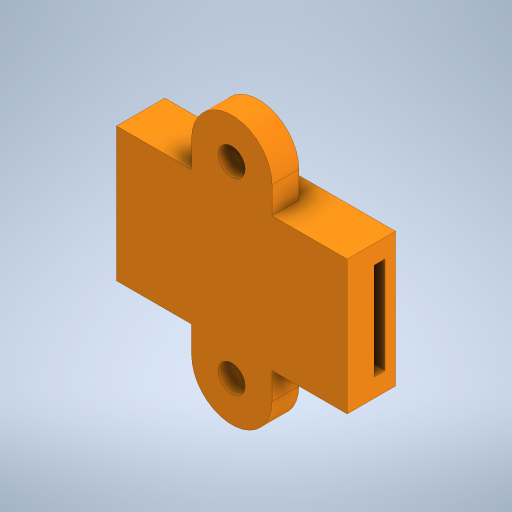
# Autodesk Inventor part: RelayBracket
Saved by Autodesk Inventor 2023 (Build 270158000, 158)
## iProperties
Created: 2022-09-10
Part Number: RelayBracket
Material: Generic
Document SubType Name: Modeling
Designer: Nathann
Density: 1 g/cm^3
Appearance: Orange
Author: Nathann
Autodesk Inventor part; units mm, degrees
ref_plane "YZ Plane" through (0, 0, 0) normal (1, 0, 0) x (0, 1, 0)
ref_plane "XZ Plane" through (0, 0, 0) normal (0, 1, 0) x (-1, 0, 0)
ref_plane "XY Plane" through (0, 0, 0) normal (0, 0, 1) x (1, 0, 0)
sketch "Sketch1" plane through (0, 0, 0) normal (0, 0, 1) x (1, 0, 0)
  line L0 (24.4382, -12.9356) -> (-18.5618, -12.9356)
  line L1 (-18.5618, -12.9356) -> (-18.5618, 12.0644)
  line L2 (-18.5618, 12.0644) -> (24.4382, 12.0644)
  line L3 (24.4382, 12.0644) -> (24.4382, -12.9356)
  line L4 (-4.5618, -12.9356) -> (10.4382, -12.9356)
  line L5 (10.4382, -12.9356) -> (10.4382, -17.9356)
  line L6 (10.4382, -17.9356) -> (-4.5618, -17.9356)
  line L7 (-4.5618, -17.9356) -> (-4.5618, -12.9356)
  line L8 (-4.5618, 12.0644) -> (10.4382, 12.0644)
  line L9 (10.4382, 12.0644) -> (10.4382, 17.0644)
  line L10 (10.4382, 17.0644) -> (-4.5618, 17.0644)
  line L11 (-4.5618, 17.0644) -> (-4.5618, 12.0644)
  circle A0 centre (2.9382, -17.9356) radius 7.5
  circle A1 centre (2.9382, 17.0644) radius 7.5
  circle A2 centre (2.9382, -17.9356) radius 2.5
  circle A3 centre (2.9382, 17.0644) radius 2.5
  point P0 (0, 0)
  point P1 (-4.5618, -17.9356)
  dimension "d0" = 43
  dimension "d1" = 25
  dimension "d2" = 15
  dimension "d3" = 15
  dimension "d4" = 21.5
  dimension "d5" = 21.5
  dimension "d6" = 5
  dimension "d7" = 5
  dimension "d8" = 5
  dimension "d9" = 5
  constraints: 24 end point, 6 parallel, 3 horizontal, 3 perpendicular, 2 centre point, 2 coincident, 2 midpoint, 2 point on line, 6 other
  measures "d0" distance of L0.start L0.end
  measures "d1" distance of L2.end L0.start
  measures "d2" distance between parallel lines of L7 L5
  measures "d3" distance between parallel lines of L11 L9
  measures "d4" distance from line of L1 point (2.938, 17.064)
  measures "d5" distance from line of L1 point (2.938, -17.936)
  measures "d6" distance of L8.end L9.end
  measures "d7" distance of L4.end L5.end
  measures "d8" diameter of A2
  measures "d9" diameter of A3
extrude "Extrusion1" add sketch "Sketch1" along normal blind 5 contours L0 A0 L1 L2 A1 L3 | L5 A0 L0 | A0 L6 A2 L0 | L0 A0 | A0 L6 A2 | L2 A1 L9 | A0 L7 L0 | A1 L2 | L2 A1 L10 A3 | L10 A3 A1 | L2 L11 A1
sketch "Sketch2" plane through (0, 0, 0) normal (0, 0, -1) x (-1, 0, 0)
  line L0 (18.5618, 12.0644) -> (18.5618, -12.9356) projected
  line L1 (-24.4382, -12.9356) -> (-24.4382, 12.0644) projected
  line L2 (18.5618, -12.9356) -> (-24.4382, -12.9356)
  line L3 (-24.4382, -12.9356) -> (-24.4382, -9.4356)
  line L4 (-24.4382, -9.4356) -> (18.5618, -9.4356)
  line L5 (18.5618, -9.4356) -> (18.5618, -12.9356)
  line L6 (-24.4382, 12.0644) -> (18.5618, 12.0644)
  line L7 (18.5618, 12.0644) -> (18.5618, 8.5644)
  line L8 (18.5618, 8.5644) -> (-24.4382, 8.5644)
  line L9 (-24.4382, 8.5644) -> (-24.4382, 12.0644)
  point P0 (0, 0)
  point P1 (-24.4382, 8.5644)
  point P2 (18.5618, -9.4356)
  dimension "d12" = 3.5
  dimension "d13" = 3.5
  constraints: 16 end point, 4 parallel, 2 horizontal, 2 perpendicular, 2 point on line
  measures "d12" distance between parallel lines of L2 L4
  measures "d13" distance between parallel lines of L6 L8
extrude "Extrusion2" add sketch "Sketch2" along normal blind 2 contours L0 L8 L1 L6 | L0 L2 L1 L4
sketch "Sketch3" plane through (0, 0, -2) normal (0, 0, -1) x (-1, 0, 0)
  line L0 (-24.4382, -12.9356) -> (18.5618, -12.9356) projected
  line L1 (-24.4382, -9.4356) -> (-24.4382, 8.5644) projected
  line L2 (18.5618, -12.9356) -> (-24.4382, -12.9356)
  line L3 (-24.4382, -12.9356) -> (-24.4382, -8.9356)
  line L4 (-24.4382, -8.9356) -> (18.5618, -8.9356)
  line L5 (18.5618, -8.9356) -> (18.5618, -12.9356)
  line L6 (-24.4382, 12.0644) -> (18.5618, 12.0644)
  line L7 (18.5618, 12.0644) -> (18.5618, 8.0644)
  line L8 (18.5618, 8.0644) -> (-24.4382, 8.0644)
  line L9 (-24.4382, 8.0644) -> (-24.4382, 12.0644)
  line L10 (-24.4382, -8.9356) -> (-22.4382, -8.9356)
  line L11 (-22.4382, -8.9356) -> (-22.4382, 8.0644)
  line L12 (-22.4382, 8.0644) -> (-24.4382, 8.0644)
  line L13 (-24.4382, 8.0644) -> (-24.4382, -8.9356)
  line L14 (-22.4382, -3.6663) -> (-20.4382, -3.6663)
  line L15 (-20.4382, -3.6663) -> (-20.4382, 2.486)
  line L16 (-20.4382, 2.486) -> (-22.4382, 2.486)
  line L17 (-22.4382, 2.486) -> (-22.4382, -3.6663)
  line L18 (18.5618, 12.0644) -> (-24.4382, 12.0644) projected
  point P0 (0, 0)
  dimension "d16" = 4
  dimension "d17" = 4
  dimension "d18" = 0
  dimension "d19" = 2
  dimension "d20" = 2
  constraints: 32 end point, 8 parallel, 5 point on line, 4 horizontal, 4 perpendicular
  measures "d16" distance of L4.end L0.end
  measures "d17" distance of L6.end L7.end
  measures "d18" distance between parallel lines of L18 L6
  measures "d19" distance between parallel lines of L17 L15
  measures "d20" distance between parallel lines of L1 L11
extrude "Extrusion3" add sketch "Sketch3" along normal blind 2
equation "\"d4\" = 0.5 * d0"
equation "\"d5\" = d4"
equation "\"d9\" = d8"
equation "\"d12\" = d13"
body "Solid1"
